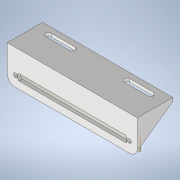
# Autodesk Inventor part: Halterung_Winkel
Saved by Autodesk Inventor 2022.2 (Build 262287010, 287A)
## iProperties
Created: 2024-04-03
Part Number: Halterung_Winkel
Material: Generisch
Document SubType Name: Modeling
Designer: ppovolni
Density: 1 g/cm^3
Appearance: Vorgabe
Author: ppovolni
Autodesk Inventor part; units mm, degrees
ref_plane "YZ Plane" through (0, 0, 0) normal (1, 0, 0) x (0, 1, 0)
ref_plane "XZ Plane" through (0, 0, 0) normal (0, 1, 0) x (-1, 0, 0)
ref_plane "XY Plane" through (0, 0, 0) normal (0, 0, 1) x (1, 0, 0)
ref_plane "Arbeitsebene1" through (0, 0, 0) normal (0, 0, 1) x (1, 0, 0)
sketch "Skizze1" plane through (0, 0, 0) normal (0, 0, 1) x (1, 0, 0)
  spline S0 degree 3 poles (34.5, 0) (34.4922, -0.0784) (34.4879, -0.2047) (34.5533, -0.4702) (34.6001, -0.5784) (34.7323, -0.7826) (34.8194, -0.8753) (34.994, -1.0048) (35.1117, -1.0785) (35.3805, -1.1607) (35.4924, -1.1779) (35.724, -1.1797) (35.8424, -1.1625) (35.9562, -1.1277) knots 0 0 0 0 0.253865 0.253865 0.443826 0.443826 0.648627 0.648627 0.796581 0.796581 0.895512 0.895512 1 1 1 1 construction
  circle A0 centre (35.5, 0) radius 1 construction
  circle A1 centre (-35.5, 0) radius 1 construction
  line L0 (-36.5594, -4.5) -> (36.5594, -4.5) construction
  line L1 (37.5, -3.5594) -> (37.5, 3.5594) construction
  line L2 (-36.5594, 4.5) -> (36.5594, 4.5) construction
  line L3 (-37.5, -3.5594) -> (-37.5, 3.5594) construction
  line L4 (-36.95, 3.5319) -> (-36.95, -3.5319) construction
  arc A2 (-36.5319, -3.95) -> (-36.95, -3.5319) centre (-37.1503, -4.1503) ccw construction
  line L5 (-36.5319, -3.95) -> (36.5319, -3.95) construction
  arc A3 (36.95, -3.5319) -> (36.5319, -3.95) centre (37.1503, -4.1503) ccw construction
  line L6 (36.95, 3.5319) -> (36.95, -3.5319) construction
  arc A4 (36.5319, 3.95) -> (36.95, 3.5319) centre (37.1503, 4.1503) ccw construction
  line L7 (-36.5319, 3.95) -> (36.5319, 3.95) construction
  arc A5 (-36.95, 3.5319) -> (-36.5319, 3.95) centre (-37.1503, 4.1503) ccw construction
  spline S1 degree 3 poles (-36.5, 0) (-36.5078, -0.0784) (-36.5121, -0.2047) (-36.4467, -0.4702) (-36.3999, -0.5784) (-36.2677, -0.7826) (-36.1806, -0.8753) (-36.006, -1.0048) (-35.8883, -1.0785) (-35.6195, -1.1607) (-35.5076, -1.1779) (-35.276, -1.1797) (-35.1576, -1.1625) (-35.0438, -1.1277) knots 0 0 0 0 0.253865 0.253865 0.443826 0.443826 0.648627 0.648627 0.796581 0.796581 0.895512 0.895512 1 1 1 1 construction
  arc A6 (-35.5, 1) -> (-36.5, 0) centre (-35.5, 0) ccw construction
  spline S2 degree 3 poles (-34.3787, -0.4718) (-34.3466, -0.3696) (-34.3281, -0.2637) (-34.32, -0.0752) (-34.3224, 0.0413) (-34.3918, 0.3184) (-34.4553, 0.4524) (-34.6302, 0.687) (-34.7395, 0.7855) (-34.9556, 0.9143) (-35.0636, 0.9616) (-35.2916, 1.0075) (-35.3964, 1.012) (-35.5, 1) knots 0 0 0 0 0.226159 0.226159 0.39844 0.39844 0.580791 0.580791 0.761736 0.761736 0.893125 0.893125 1 1 1 1 construction
  arc A7 (-35.0438, -1.1277) -> (-34.3787, -0.4718) centre (-35.5, 0) ccw construction
  spline S3 degree 3 poles (34.5, 0) (34.4922, -0.0784) (34.4879, -0.2047) (34.5533, -0.4702) (34.6001, -0.5784) (34.7323, -0.7826) (34.8194, -0.8753) (34.994, -1.0048) (35.1117, -1.0785) (35.3805, -1.1607) (35.4924, -1.1779) (35.724, -1.1797) (35.8424, -1.1625) (35.9562, -1.1277) knots 0 0 0 0 0.253865 0.253865 0.443826 0.443826 0.648627 0.648627 0.796581 0.796581 0.895512 0.895512 1 1 1 1 construction
  arc A8 (35.5, 1) -> (34.5, 0) centre (35.5, 0) ccw construction
  spline S4 degree 3 poles (36.6213, -0.4718) (36.6534, -0.3696) (36.6719, -0.2637) (36.68, -0.0752) (36.6776, 0.0413) (36.6082, 0.3184) (36.5447, 0.4524) (36.3698, 0.687) (36.2605, 0.7855) (36.0444, 0.9143) (35.9364, 0.9616) (35.7084, 1.0075) (35.6036, 1.012) (35.5, 1) knots 0 0 0 0 0.226159 0.226159 0.39844 0.39844 0.580791 0.580791 0.761736 0.761736 0.893125 0.893125 1 1 1 1 construction
  arc A9 (35.9562, -1.1277) -> (36.6213, -0.4718) centre (35.5, 0) ccw construction
  line L8 (-33.5, 1) -> (-33.5, -1) construction
  arc A10 (-33, 1.5) -> (-33.5, 1) centre (-33, 1) ccw construction
  line L9 (33, 1.5) -> (-33, 1.5) construction
  arc A11 (33.5, 1) -> (33, 1.5) centre (33, 1) ccw construction
  line L10 (33.5, -1) -> (33.5, 1) construction
  arc A12 (33, -1.5) -> (33.5, -1) centre (33, -1) ccw construction
  line L11 (-33, -1.5) -> (33, -1.5) construction
  arc A13 (-33.5, -1) -> (-33, -1.5) centre (-33, -1) ccw construction
  line L12 (40.5, -6.5) -> (-40.5, -6.5)
  line L13 (-40.5, -6.5) -> (-40.5, 15)
  line L14 (-40.5, 15) -> (40.5, 15)
  line L15 (40.5, 15) -> (40.5, -6.5)
  circle A14 centre (35.5, 0) radius 1.25
  circle A15 centre (-35.5, 0) radius 1.25
  arc A16 (33, -2) -> (34, -1) centre (33, -1) ccw
  line L16 (34, -1) -> (34, 1)
  arc A17 (34, 1) -> (33, 2) centre (33, 1) ccw
  line L17 (33, 2) -> (-33, 2)
  arc A18 (-33, 2) -> (-34, 1) centre (-33, 1) ccw
  line L18 (-34, 1) -> (-34, -1)
  arc A19 (-34, -1) -> (-33, -2) centre (-33, -1) ccw
  line L19 (-33, -2) -> (33, -2)
  point P0 (0, 0)
  dimension "d0" = 5
  dimension "d1" = 5
  dimension "d2" = 2
  dimension "d3" = 15
  dimension "d4" = 2.5
  dimension "d5" = 2.5
  constraints: 16 end point, 8 point on circle, 6 centre point, 2 coincident, 2 parallel, 1 horizontal, 1 perpendicular, 7 other
  measures "d0" distance from line of L15 A0.centre
  measures "d1" distance from line of A1.centre L13
  measures "d2" distance between parallel lines of L0 L12
  measures "d3" distance from line of L14 A0.centre
  measures "d4" diameter of A14
  measures "d5" diameter of A15
extrude "Extrusion1" add sketch "Skizze1" along normal blind 2
fillet "Rundung1" radius 5 2 edges at (40.5, -6.5, 1) (-40.5, -6.5, 1)
sketch "Skizze2" plane through (0, 0, 0) normal (0, 0, -1) x (-1, 0, 0)
  line L0 (-40.5, 15) -> (40.5, 15) construction
  line L1 (40.5, 15) -> (40.5, -1.5) construction
  line L2 (-40.5, -1.5) -> (-40.5, 15) construction
  line L3 (40.5, 15) -> (-40.5, 15)
  line L4 (-40.5, 15) -> (-40.5, 13)
  line L5 (-40.5, 13) -> (40.5, 13)
  line L6 (40.5, 13) -> (40.5, 15)
  point P0 (0, 0)
  dimension "d9" = 2
  constraints: 8 end point, 2 parallel, 1 horizontal, 1 perpendicular, 1 point on line
  measures "d9" distance between parallel lines of L0 L5
extrude "Extrusion2" add sketch "Skizze2" along normal blind 20
sketch "Skizze3" plane through (40.5, -1.5, 2) normal (1, 0, 0) x (0, 0, -1)
  line L0 (2, 0) -> (0, 0) construction
  line L1 (2, 0) -> (2, 14.5) projected
  line L2 (2, 14.5) -> (22, 14.5) projected
  line L3 (22, 16.5) -> (22, 14.5) construction
  line L4 (0, 16.5) -> (22, 16.5) construction
  line L5 (0, 0) -> (0, 16.5) construction
  line L6 (2, 0) -> (22, 14.5)
  point P0 (2, 1.5)
  constraints: 2 end point
extrude "Extrusion3" add sketch "Skizze3" against normal blind 1
sketch "Skizze4" plane through (-40.5, -1.5, 2) normal (-1, 0, 0) x (0, 0, 1)
  line L0 (-22, 14.5) -> (-2, 14.5) projected
  line L1 (-22, 14.5) -> (-2, 0) projected
  line L2 (-2, 14.5) -> (-2, 0) projected
  point P0 (-2, 1.5)
extrude "Extrusion4" add sketch "Skizze4" against normal blind 1
sketch "Skizze5" plane through (39.5, 13, -20) normal (0, -1, 0) x (1, 0, 0)
  line L0 (-0.5716, 5) -> (-194.7619, 5) construction
  line L1 (-7.5, 5) -> (-22.5, 5) construction
  line L2 (-7.5, 6.75) -> (-22.5, 6.75)
  line L3 (-22.5, 3.25) -> (-7.5, 3.25)
  arc A0 (-7.5, 3.25) -> (-7.5, 6.75) centre (-7.5, 5) ccw
  arc A1 (-22.5, 6.75) -> (-22.5, 3.25) centre (-22.5, 5) ccw
  line L4 (-56.5, 5) -> (-71.5, 5) construction
  line L5 (-56.5, 6.75) -> (-71.5, 6.75)
  line L6 (-71.5, 3.25) -> (-56.5, 3.25)
  arc A2 (-56.5, 3.25) -> (-56.5, 6.75) centre (-56.5, 5) ccw
  arc A3 (-71.5, 6.75) -> (-71.5, 3.25) centre (-71.5, 5) ccw
  line L7 (0, 0) -> (-79, 0) projected
  line L8 (0, 0) -> (0, 20) projected
  line L9 (-79, 20) -> (-79, 0) projected
  point P0 (-39.5, 20)
  point P1 (-15, 5)
  point P2 (-64, 5)
  dimension "d16" = 3.5
  dimension "d17" = 15
  dimension "d18" = 5
  dimension "d19" = 15
  dimension "d20" = 15
  constraints: 18 end point, 8 point on circle, 8 tangent, 4 centre point, 4 point on line, 2 midpoint, 2 parallel, 1 collinear, 1 equal radius
  measures "d16" distance between parallel lines of L2 L3
  measures "d17" distance of L3.start L3.end
  measures "d18" distance between parallel lines of L0 L7
  measures "d19" distance from line of L8 point (-15, 5)
  measures "d20" distance from line of L9 point (-64, 5)
extrude "Extrusion5" cut sketch "Skizze5" against normal through all
